Camera Mast Old (Autodesk Fusion 360 design; units mm, degrees)
Autodesk Fusion 360 part; units mm, degrees
sketch "Sketch1" plane through (0, 0, 0) normal (0, 0, 1) x (1, 0, 0) in component "Arm Cam"
  circle A0 centre (0, 0) radius 14.75
  circle A1 centre (0, 0) radius 11.75
  dimension "d322" = 29.5
  dimension "d323" = -3
  dimension "d395" = 23.5
  constraint coincident A0.centre A1.centre
  measures "d322" diameter of A0
  measures "d395" diameter of A1
extrude "Extrude1" add sketch "Sketch1" along normal blind 67.1 makes body 1 in component "Arm Cam"
sketch "Sketch5" plane through (0, 0, 67.1) normal (0, 0, 1) x (-1, 0, 0) in component "Arm Cam"
  circle A0 centre (0, 0) radius 11.75
  circle A1 centre (0, 0) radius 14.75
  circle A2 centre (0, 0) radius 14.75
  constraint concentric A0 A2
ref_plane "WorkPlane2" through (0, 0, 75.5) normal (0, 0, 1) x (1, 0, 0) in component "Arm Cam"
sketch "Sketch4" plane through (-143.4796, -223.0695, 75.5) normal (0, 0, 1) x (1, 0, 0) in component "Arm Cam"
  circle A0 centre (143.4796, 223.0695) radius 14.75
  circle A1 centre (143.4796, 223.0695) radius 12.15
  point P0 (143.4796, 223.0695)
  dimension "d330" = 29.5
  dimension "d334" = 24.3
  constraint concentric A0 A1
  constraint coincident P0 A0.centre
  measures "d330" diameter of A0
  measures "d334" diameter of A1
loft "Loft2" add profiles "Sketch5", "Sketch4" section 1 section 2 contours A1 bodies 1 in component "Arm Cam"
extrude "Extrude4" add sketch "Sketch4" along normal blind 7.4 contours A0 | A1 bodies 1 in component "Arm Cam"
sketch "Sketch7" plane through (0, 0, 82.9) normal (0, 0, 1) x (-1, 0, 0) in component "Arm Cam"
  circle A0 centre (0, 0) radius 14.75
  circle A1 centre (0, 0) radius 16.75
  dimension "d339" = 33.5
  constraint concentric A0 A1
  measures "d339" diameter of A1
extrude "Extrude5" add sketch "Sketch7" along normal blind 3.35 contours A0 | A1 bodies 1 in component "Arm Cam"
ref_plane "WorkPlane3" through (0, 0, 89.15) normal (0, 0, 1) x (-1, 0, 0) in component "Arm Cam"
sketch "Sketch8" plane through (-143.4796, -223.0695, 89.15) normal (0, 0, 1) x (1, 0, 0) in component "Arm Cam"
  circle A0 centre (143.4796, 223.0695) radius 13.75
  point P0 (143.4796, 223.0695)
  dimension "d341" = 27.5
  constraint coincident P0 A0.centre
  measures "d341" diameter of A0
extrude "Extrude6" add sketch "Sketch8" along normal blind 7.7 separate body makes body 2 in component "Arm Cam"
loft "Loft3" add section 1 face at (-0.9963, -4.3652, 86.25) section 2 face at (-1.0199, 5.8346, 89.15) on bodies 1 2 bodies 1 2 in component "Arm Cam"
sketch "Sketch9" plane through (0, 0, 96.85) normal (0, 0, 1) x (-1, 0, 0) in component "Arm Cam"
  circle A0 centre (0, 0) radius 13.75
  circle A1 centre (0, 0) radius 33
  dimension "d344" = 66
  dimension "d351" = 27.5
  constraint concentric A0 A1
  measures "d344" diameter of A1
  measures "d351" diameter of A0
extrude "Extrude7" add sketch "Sketch9" along normal blind 17 contours A0 | A1 bodies 1 in component "Arm Cam"
sketch "Sketch10" plane through (0, 0, 113.85) normal (0, 0, 1) x (-1, 0, 0) in component "Arm Cam"
  circle A0 centre (0, 0) radius 33
  line L0 (-17.6, 17.6) -> (17.6, 17.6)
  line L1 (17.6, 17.6) -> (17.6, -17.6)
  line L2 (17.6, -17.6) -> (-17.6, -17.6)
  line L3 (-17.6, -17.6) -> (-17.6, 17.6)
  line L4 (-17.6, 17.6) -> (17.6, -17.6) construction
  line L5 (17.6, 17.6) -> (-17.6, -17.6) construction
  circle A1 centre (0, 0) radius 7.5
  line L6 (-17.6, 3) -> (17.6, 3)
  line L7 (17.6, 3) -> (17.6, -3)
  line L8 (17.6, -3) -> (-17.6, -3)
  line L9 (-17.6, -3) -> (-17.6, 3)
  line L10 (-17.6, 3) -> (17.6, -3) construction
  line L11 (17.6, 3) -> (-17.6, -3) construction
  line L12 (-22.5, 22.5) -> (22.5, 22.5) construction
  line L13 (22.5, 22.5) -> (22.5, -22.5) construction
  line L14 (22.5, -22.5) -> (-22.5, -22.5) construction
  line L15 (-22.5, -22.5) -> (-22.5, 22.5) construction
  line L16 (-22.5, 22.5) -> (22.5, -22.5) construction
  line L17 (22.5, 22.5) -> (-22.5, -22.5) construction
  circle A2 centre (22.5, 0) radius 0.75
  circle A3 centre (0, -22.5) radius 0.75
  circle A4 centre (-22.5, 0) radius 0.75
  circle A5 centre (0, 22.5) radius 0.75
  dimension "d347" = 35.2
  dimension "d348" = 35.2
  dimension "d352" = 15
  dimension "d354" = 6
  dimension "d357" = 45
  dimension "d358" = 45
  dimension "d359" = 1.5
  dimension "d360" = 1.5
  dimension "d361" = 1.5
  dimension "d362" = 1.5
  constraint perpendicular L0 L1
  constraint parallel L0 L2
  constraint parallel L1 L3
  constraint horizontal L0
  constraint coincident L4 A0.centre
  constraint coincident L5 A0.centre
  constraint coincident A0.centre A1.centre
  constraint concentric A0 A1
  constraint perpendicular L6 L7
  constraint parallel L6 L8
  constraint parallel L7 L9
  constraint horizontal L6
  constraint coincident L3 L6.start
  constraint coincident L10 A0.centre
  constraint coincident L11 A0.centre
  constraint perpendicular L12 L13
  constraint parallel L12 L14
  constraint parallel L13 L15
  constraint horizontal L12
  constraint coincident L16 A0.centre
  constraint coincident L17 A0.centre
  constraint midpoint L13 A2.centre
  constraint midpoint L14 A3.centre
  constraint midpoint L15 A4.centre
  constraint midpoint L12 A5.centre
  measures "d347" distance of L0.end L1.end
  measures "d348" distance of L1.end L2.end
  measures "d352" diameter of A1
  measures "d354" distance of L6.end L7.end
  measures "d357" distance of L12.end L13.end
  measures "d358" distance of L13.end L14.end
  measures "d359" diameter of A2
  measures "d360" diameter of A3
  measures "d361" diameter of A4
  measures "d362" diameter of A5
extrude "Extrude8" cut sketch "Sketch10" against normal blind 14 contours L0 L1 L3 A1 L6 | L3 A1 L6 L8 L9 | L1 A1 L6 L7 L8 | L1 L2 L3 A1 L8 | A1 L6 L8 | A1 L6 | A1 L8 bodies 1 in component "Arm Cam"
extrude "Extrude9" cut sketch "Sketch10" against normal through all contours A1 L6 L8 | A1 L6 | A1 L8 bodies 1 in component "Arm Cam"
extrude "Extrude10" cut sketch "Sketch10" against normal blind 15 contours L3 A1 L6 L8 L9 | L1 A1 L6 L7 L8 bodies 1 in component "Arm Cam"
extrude "Extrude11" cut sketch "Sketch10" against normal blind 10 contours A2 | A3 | A4 | A5 bodies 1 in component "Arm Cam"
component "Arm Cam" placed x (1, 0, 0) y (0, 1, 0) z (0, 0, 1) at (0, 0, 0)
equation "Trous_Vis_diam2 = 2.2 mm"
named bodies: "Bras"
